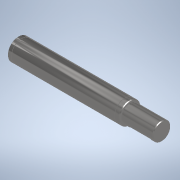
# Autodesk Inventor part: KZBN17-113-P14-LA25-TC4-TB4-KB21-HB50-ZA3-HA18-AA120_b
Saved by Autodesk Inventor 2021.3 (Build 253353000, 353)
## iProperties
Part Number: KZBN17-113-P14-LA25-TC4-TB4-KB21-HB50-ZA3-HA18-AA120_b
Material: Stainless Steel
Catalog Web Link: www.cadenas.de
Description: KZBE, KZBN, KZBC, KZBP, KZBF_b-Driving Shaft - One End Stepped -
Vendor: MISUMI
Document SubType Name: Modeling
Designer: partserver
Manufacturer: MISUMI
Mass: 181.625 g
Surface Area: 66.9686 cm^2
Volume: 22.7031 cm^3
Density: 8 g/cm^3
Appearance: Semi-Polished
Category: PARTsolutions
Company: MISUMI
PSOL_IDENT_0: {$CADENAS_DATA\23d-libs\misumi\metric\11_rotary_shafts\11_components\kzbc\kzbc.prj},738 {VTYP=3D},{N
PSOL_IDENT_1: B=KZBN17-113-P14-LA25-TC4-TB4-KB21-HB50-ZA3-HA18-AA120_b},{LINA=KZBN17-113-P14-LA25-TC4-TB4-KB21-HB5
PSOL_IDENT_2: 0-ZA3-HA18-AA120},{NN=KZBE, KZBN, KZBC, KZBP, KZBF_b},{DATE=27.07.2021 05:05:17},{GEOMDATE=01.11.201
PSOL_IDENT_3: 9 08:10:50},{VERSION=},{LINEID=60},{WBVAR=TS,HARD,ST,L,P,LA,ALT1,MA,MSA,MMA,ALT4,MD,MSD,MMD,ALT2,MB,
PSOL_IDENT_4: MSB,MMB,ALT5,NA,NBALT5,ALT7,TA,ALT6,TC,TB,ALT9,KA,HAALT9,ALT10,KB,HBALT10,KC,HCALT10,ALT12,ZA,HAALT1
PSOL_IDENT_5: 2,AAALT12,ALT13,ZB,HBALT13,ABALT13,ZC,HCALT13,ACALT13,ALT15,SA,ALT16,SC,ALT18,WA,GA,AAALT18,ALT19,WB
PSOL_IDENT_6: ,GB,ABALT19,WC,GC,ACALT19},{WBNUMERIC=L,P,LA,MA,MSA,MMA,MD,MSD,MMD,MB,MSB,MMB,TA,TC,TB,KA,HAALT9,KB,
PSOL_IDENT_7: HBALT10,KC,HCALT10,ZA,HAALT12,AAALT12,ZB,HBALT13,ABALT13,ZC,HCALT13,ACALT13,SA,SC,WA,GA,AAALT18,WB,G
PSOL_IDENT_8: B,ABALT19,WC,GC,ACALT19}  {NB=KZBN17-113-P14-LA25-TC4-TB4-KB21-HB50-ZA3-HA18-AA120_b},{LINA=KZBN17-1
PSOL_IDENT_9: 13-P14-LA25-TC4-TB4-KB21-HB50-ZA3-HA18-AA120},{KT=DUMMY},{PN=KZBN17-113-P14-LA25-TC4-TB4-KB21-HB50-Z
PSOL_IDENT_10: A3-HA18-AA120},{TYPE=KZBN},{D=17},{TS=h6},{TSALG= 'h7','h7','h6','h6' },{HARD=-},{HARDALG= '-','-','
PSOL_IDENT_11: IHSH50','Induction Hardened Surface Hardness 50HRC' },{ST=-},{STALG= '-','-','BO','Black Oxide','ENP'
PSOL_IDENT_12: ,'Electroless Nickel Plating'},{L=113.0},{LALG=[100:400/0.5]},{P=14},{PALG=[10:16/1]},{PMIN=10},{PMA
PSOL_IDENT_13: X=16},{LA=25.0},{LAALG=[10:56.5/0.5]},{LAMIN=10.0},{LAMAX=56.5},{CIFCC=0.5},{CIFR=0.0},{ALT1=},{ALT1
PSOL_IDENT_14: ALG= '','Not applicable' },{ALT1PN=},{MA=0},{MAALG=[0]},{MAMIN=0},{MAMAX=0},{MSA=0},{MSAALG=[0]},{MS
PSOL_IDENT_15: AMIN=0},{MSAMAX=0},{MMA=0},{MMAALG=[0]},{MMAMIN=0},{MMAMAX=0},{MALT1=0},{APITCH=0.00},{ALT4=},{ALT4A
PSOL_IDENT_16: LG= '','w/o Shaft End D Threaded Left End','MSD','with MSD (Fine (Standard) JIS 6h (Class 2))','MMD'
PSOL_IDENT_17: ,'with MMD (Fine (Precision) JIS 4h (Class 1))' },{ALT4PN=},{MD=0},{MDALG=[0]},{MDMIN=0},{MDMAX=0},{
PSOL_IDENT_18: MSD=0},{MSDALG=[0]},{MSDMIN=0},{MSDMAX=0},{MMD=0},{MMDALG=[0]},{MMDMIN=0},{MMDMAX=0},{MALT4=0},{DPIT
PSOL_IDENT_19: CH=0.00},{MDPITCH=0},{MSDPITCH=1},{ALT2=},{ALT2ALG= '','w/o Shaft End D Threaded Right End','MSB','w
PSOL_IDENT_20: ith MSB (Fine (Standard) JIS 6h (Class 2))','MMB','with MMB (Fine (Precision) JIS 4h (Class 1))' },{
PSOL_IDENT_21: ALT2PN=},{MB=0},{MBALG=[0]},{MBMIN=0},{MBMAX=0},{MSB=0},{MSBALG=[0]},{MSBMIN=0},{MSBMAX=0},{MMB=0},{
PSOL_IDENT_22: MMBALG=[0]},{MMBMIN=0},{MMBMAX=0},{MALT2=0},{BPITCH=0.00},{ALT5=},{ALT5ALG= '','w/o Tapped Ends','NA'
PSOL_IDENT_23: ,'with NA (Tapped Left End)','NB','with NB (Tapped Right End)','NANB','with NA + NB (Tapped Both End
PSOL_IDENT_24: s)' },{ALT5PN=},{NA=0},{NAALG= '0','N/A' },{NAMAX=10},{NA1=0},{NAL=0},{PITCHA=0},{NBALT5=0},{NBALT5A
PSOL_IDENT_25: LG= '0','N/A' },{NBMAX=12},{NBMAX1=24},{NBMAX2=12},{NBMAX3=12},{NBMAX4=0},{NB1=0},{NBL=0},{PITCHB=0}
PSOL_IDENT_26: ,{CIFNA=0},{ALT7=},{ALT7ALG=  '','w/o Shaft End P Retaining Ring Groove','TA','with TA (Shaft End P
PSOL_IDENT_27: Retaining Ring Groove)' },{ALT7PN=},{TA=0},{TAALG=[0]},{TAMIN=4},{TAMAX=22},{DDALT7=0.0},{MMALT7=0.0
PSOL_IDENT_28: 0},{ALT6=TCTB},{ALT6ALG=  '','w/o Shaft End D Retaining Ring Grooves','TC','with TC (Shaft End D Ret
PSOL_IDENT_29: aining Ring Groove Left End)','TB','with TB (Shaft End D Retaining Ring Groove Right End)','TCTB','w
PSOL_IDENT_30: ith TC + TB (Shaft End D Retaining Ring Grooves Both Ends)' },{ALT6PN=-TC4-TB4},{TC=4},{TCALG=[4:82/
PSOL_IDENT_31: 1]},{TCMIN=4},{TCMAX=82},{TB=4},{TBALG=[4:86/1]},{TBMIN=4},{TBMAX=86},{DDALT6=16.2},{MMALT6=1.15},{A
PSOL_IDENT_32: LT9=},{ALT9ALG= '','w/o Shaft End P Key Groove','KA','with KA (Shaft End P Key Groove)' },{ALT9PN=},
PSOL_IDENT_33: {KA=0},{KAALG=[0]},{KAMIN=0},{KAMAX=18},{HAALT9=0},{HAALT9ALG=[0]},{HAALT9MIN=5},{HAALT9MAX=23},{PBB=
PSOL_IDENT_34: 5},{PTT=3.0},{ALT10=KB},{ALT10ALG= '','w/o Shaft End D Key Grooves','KB','with KB (Shaft End D Key G
PSOL_IDENT_35: roove)','KBKC','with KB + KC (Shaft End D Two Key Grooves)' },{ALT10PN=-KB21-HB50},{KB=21},{KBALG=[2
PSOL_IDENT_36: :83/1]},{KBMIN=2},{KBMAX1=83},{KBMAX2=76},{HBALT10=50},{HBALT10ALG=[5:67/1]},{HBALT10MIN=5},{HBALT10
PSOL_IDENT_37: MAX1=67},{HBALT10MAX2=60},{KC=0},{KCALG=[0]},{KCMIN=73},{KCMAX=83},{HCALT10=0},{HCALT10ALG=[0]},{HCA
PSOL_IDENT_38: LT10MIN=5},{HCALT10MAX=88},{DBB=5},{DTT=3.0},{ALT12=ZA},{ALT12ALG= '','w/o Shaft End P Key Groove +
PSOL_IDENT_39: Set Screw Flat','ZA','with ZA (Shaft End P Key Groove + Set Screw Flat)' },{ALT12PN=-ZA3-HA18-AA120}
PSOL_IDENT_40: ,{ZA=3},{ZAALG=[0:18/1]},{ZAMIN=0},{ZAMAX=18},{HAALT12=18},{HAALT12ALG=[5:20/1]},{HAALT12MIN=5},{HAA
PSOL_IDENT_41: LT12MAX=20},{AAALT12=120},{AAALT12ALG=[60:300/30]},{PH=1},{ALT13=},{ALT13ALG= '','Not applicable' },
PSOL_IDENT_42: {ALT13PN=},{ZB=0},{ZBALG=[0]},{ZBMIN=2},{ZBMAX1=83},{ZBMAX2=76},{HBALT13=0},{HBALT13ALG=[0]},{HBALT1
PSOL_IDENT_43: 3MIN=5},{HBALT13MAX1=88},{HBALT13MAX2=81},{ABALT13=0},{ABALT13ALG=[0]},{ZC=0},{ZCALG=[0]},{ZCMIN=2},
PSOL_IDENT_44: {ZCMAX=83},{HCALT13=0},{HCALT13ALG=[0]},{HCALT13MIN=5},{HCALT13MAX=88},{ACALT13=0},{ACALT13ALG=[0]},
PSOL_IDENT_45: {DH=0},{ALT15=},{ALT15ALG= '', 'w/o Shaft End P Wrench Flats', 'SA', 'with SA (Shaft End P Wrench Fl
PSOL_IDENT_46: ats)' },{ALT15PN=},{SA=0},{SAALG=[0]},{SAMIN=0},{SAMAX=25},{WALT15=0.0},{LLALT15=0},{ALT16=},{ALT16A
PSOL_IDENT_47: LG= '', 'w/o Shaft End D Wrench Flats', 'SC', 'with SC (Shaft End D Wrench Flats)' },{ALT16PN=},{SC=
PSOL_IDENT_48: 0},{SCALG=[0]},{SCMIN=2},{SCMAX=88},{WALT16=0},{LLALT16=0},{ALT18=},{ALT18ALG= '','Not applicable' }
PSOL_IDENT_49: ,{ALT18PN=},{WA=0},{WAALG=[0]},{WAMIN=0},{WAMAX=22},{GA=0},{GAALG=[0]},{GAMIN=3},{GAMAX=25},{AAALT18=
PSOL_IDENT_50: 0},{AAALT18ALG=[0]},{ALT19=},{ALT19ALG= '','w/o Shaft End D 2 Set Screw Flats (Angle Specified)','WB'
PSOL_IDENT_51: ,'with WB (Shaft End D 2 Set Screw Flats (Angle Specified))','WBWC','with WB + WC (Shaft End D Two 2
PSOL_IDENT_52: Set Screw Flats (Angle Specified))' },{ALT19PN=},{WB=0},{WBALG=[0]},{WBMIN=2},{WBMAX1=85},{WBMAX2=8
PSOL_IDENT_53: 0},{GB=0},{GBALG=[0]},{GBMIN=3},{GBMAX1=88},{GBMAX2=83},{ABALT19=0},{ABALT19ALG=[0]},{WC=0},{WCALG=[
PSOL_IDENT_54: 0]},{WCMIN=2},{WCMAX=85},{GC=0},{GCALG=[0]},{GCMIN=3},{GCMAX=88},{ACALT19=0},{ACALT19ALG=[0]},{ERROR
PSOL_IDENT_55: PN=},{ERRORPALT16=OK},{ERRORPALT19=OK},{ERRORALT15=OK},{ERRORALT17=OK},{ERRORALT115=OK},{ERRORALT118=
PSOL_IDENT_56: OK},{ERRORALT25=OK},{ERRORALT26=OK},{ERRORALT216=OK},{ERRORALT219=OK},{ERRORALT45=OK},{ERRORALT46=OK
PSOL_IDENT_57: },{ERRORALT416=OK},{ERRORALT419=OK},{ERRORALT59=OK},{ERRORALT510=OK},{ERRORALT512=OK},{ERRORALT513=O
PSOL_IDENT_58: K},{ERRORALT515=OK},{ERRORALT516=OK},{ERRORALT518=OK},{ERRORALT519=OK},{ERRORALT610=OK},{ERRORALT613=
PSOL_IDENT_59: OK},{ERRORALT616=OK},{ERRORALT619=OK},{ERRORALT79=OK},{ERRORALT712=OK},{ERRORALT715=OK},{ERRORALT718=
PSOL_IDENT_60: OK},{ERRORALT915=OK},{ERRORALT918=OK},{ERRORALT1016=OK},{ERRORALT1019=OK},{ERRORALT1215=OK},{ERRORAL
PSOL_IDENT_61: T1316=OK},{ERRORALT1518=OK},{ERRORALT1619=OK}
NB: KZBN17-113-P14-LA25-TC4-TB4-KB21-HB50-ZA3-HA18-AA120_b
NN: KZBE, KZBN, KZBC, KZBP, KZBF_b
NT: Driving Shaft - One End Stepped -
NBSYN: $PN._b
LINA: KZBN17-113-P14-LA25-TC4-TB4-KB21-HB50-ZA3-HA18-AA120
CATALOG: Misumi
PN: KZBN17-113-P14-LA25-TC4-TB4-KB21-HB50-ZA3-HA18-AA120
D: 17
TS: h6
HARD: -
ST: -
L: 113
P: 14
LA: 25
ALT1: Not applicable
MA: 0
MSA: 0
MMA: 0
ALT4: w/o Shaft End D Threaded Left End
MD: 0
MSD: 0
MMD: 0
ALT2: w/o Shaft End D Threaded Right End
MB: 0
MSB: 0
MMB: 0
ALT5: w/o Tapped Ends
NA: N/A
NBALT5: N/A
ALT7: w/o Shaft End P Retaining Ring Groove
TA: 0
ALT6: with TC + TB (Shaft End D Retaining Ring Grooves Both Ends)
TC: 4
TB: 4
ALT9: w/o Shaft End P Key Groove
KA: 0
HAALT9: 0
PBB: 5
PTT: 3
ALT10: with KB (Shaft End D Key Groove)
KB: 21
HBALT10: 50
KC: 0
HCALT10: 0
ALT12: with ZA (Shaft End P Key Groove + Set Screw Flat)
ZA: 3
HAALT12: 18
AAALT12: 120
PH: 1
ALT13: Not applicable
ZB: 0
HBALT13: 0
ABALT13: 0
ZC: 0
HCALT13: 0
ACALT13: 0
DH: 0
ALT15: w/o Shaft End P Wrench Flats
SA: 0
ALT16: w/o Shaft End D Wrench Flats
SC: 0
ALT18: Not applicable
WA: 0
GA: 0
AAALT18: 0
ALT19: w/o Shaft End D 2 Set Screw Flats (Angle Specified)
WB: 0
GB: 0
ABALT19: 0
WC: 0
GC: 0
ACALT19: 0
SUPPLIER: MISUMI
ARTICLENO: KZBN17-113-P14-LA25-TC4-TB4-KB21-HB50-ZA3-HA18-AA120_b
BOMINFO: KZBN17-113-P14-LA25-TC4-TB4-KB21-HB50-ZA3-HA18-AA120
CREATOR: CADENAS GmbH
Title: KZBN17-113-P14-LA25-TC4-TB4-KB21-HB50-ZA3-HA18-AA120
Author: Cadenas PARTsolutions
Comments: Driving Shaft - One End Stepped -
Autodesk Inventor part; units mm, degrees
sketch "Sketch_1" plane through (0, 0, 0) normal (0, 0, 1) x (1, 0, 0)
  line L0 (113, 0) -> (0, 0)
  line L1 (0, 0) -> (0, 6.5)
  line L2 (0, 6.5) -> (0.5, 7)
  line L3 (0.5, 7) -> (25, 7)
  line L4 (25, 7) -> (25, 8)
  line L5 (25, 8) -> (25.5, 8.5)
  line L6 (25.5, 8.5) -> (112.5, 8.5)
  line L7 (112.5, 8.5) -> (113, 8)
  line L8 (113, 8) -> (113, 0)
  line L9 (113, 0) -> (0, 0)
  constraints: 20 end point
revolve "Revolution1" add sketch "Sketch_1" angle 360 about axis through (113, 0, 0) along (1, 0, 0)
sketch "Sketch_2" plane through (0, 0, 0) normal (0, 0, 1) x (1, 0, 0)
  line L0 (50, 0) -> (-50, 0)
  line L1 (23.5, 21) -> (23.5, 6.7)
  line L2 (23.5, 6.7) -> (25, 6.7)
  line L3 (25, 6.7) -> (25, 21)
  line L4 (25, 21) -> (23.5, 21)
  constraints: 10 end point
revolve "Revolution2" cut sketch "Sketch_2" angle 360 about axis through (50, 0, 0) along (1, 0, 0)
sketch "Sketch_15" plane through (0, 0, 0) normal (0, 0, 1) x (1, 0, 0)
  line L0 (50, 0) -> (-50, 0)
  line L1 (27.85, 25.1) -> (27.85, 8.1)
  line L2 (27.85, 8.1) -> (29, 8.1)
  line L3 (29, 8.1) -> (29, 25.1)
  line L4 (29, 25.1) -> (27.85, 25.1)
  constraints: 10 end point
revolve "Revolution3" cut sketch "Sketch_15" angle 360 about axis through (50, 0, 0) along (1, 0, 0)
sketch "Sketch_16" plane through (0, 0, 0) normal (0, 0, 1) x (1, 0, 0)
  line L0 (113, 0) -> (-50, 0)
  line L1 (109, 25.1) -> (109, 8.1)
  line L2 (109, 8.1) -> (110.15, 8.1)
  line L3 (110.15, 8.1) -> (110.15, 25.1)
  line L4 (110.15, 25.1) -> (109, 25.1)
  constraints: 10 end point
revolve "Revolution4" cut sketch "Sketch_16" angle 360 about axis through (113, 0, 0) along (1, 0, 0)
sketch "Sketch_20" plane through (0, 8.5, 0) normal (0, 1, 0) x (1, 0, 0)
  arc A0 (48.5, 2.5) -> (48.5, -2.5) centre (48.5, 0) ccw
  line L0 (48.5, -2.5) -> (93.5, -2.5)
  arc A1 (93.5, -2.5) -> (93.5, 2.5) centre (93.5, 0) ccw
  line L1 (93.5, 2.5) -> (48.5, 2.5)
  constraints: 4 end point, 4 point on circle, 2 centre point
extrude "Extrusion1" cut sketch "Sketch_20" against normal blind 3
sketch "Sketch_21" plane through (0, 7, 0) normal (0, 1, 0) x (1, 0, 0)
  arc A0 (5.5, 2.5) -> (5.5, -2.5) centre (5.5, 0) ccw
  line L0 (5.5, -2.5) -> (18.5, -2.5)
  arc A1 (18.5, -2.5) -> (18.5, 2.5) centre (18.5, 0) ccw
  line L1 (18.5, 2.5) -> (5.5, 2.5)
  constraints: 4 end point, 4 point on circle, 2 centre point
extrude "Extrusion2" cut sketch "Sketch_21" against normal blind 3
sketch "Sketch_63" plane through (3, 0, 0) normal (1, 0, 0) x (0, 0, -1)
  line L0 (-13.0622, 8.6244) -> (0.9378, -15.6244)
  line L1 (0.9378, -15.6244) -> (1.8038, -15.1244)
  line L2 (1.8038, -15.1244) -> (-12.1962, 9.1244)
  line L3 (-12.1962, 9.1244) -> (-13.0622, 8.6244)
  constraints: 8 end point
extrude "Extrusion3" cut sketch "Sketch_63" along normal blind 18
ref_plane "to_c_ring_2_XY" through (28.425, 0, 0) normal (1, 0, 0) x (0, 0, 1)
ref_plane "to_c_ring_2_YZ" through (28.425, 0, 0) normal (0, 0, 1) x (0, -1, 0)
ref_plane "to_c_ring_2_ZX" through (28.425, 0, 0) normal (0, -1, 0) x (1, 0, 0)
ref_plane "to_c_ring_3_XY" through (109.575, 0, 0) normal (1, 0, 0) x (0, 0, 1)
ref_plane "to_c_ring_3_YZ" through (109.575, 0, 0) normal (0, 0, 1) x (0, -1, 0)
ref_plane "to_c_ring_3_ZX" through (109.575, 0, 0) normal (0, -1, 0) x (1, 0, 0)
body "Solid1"
